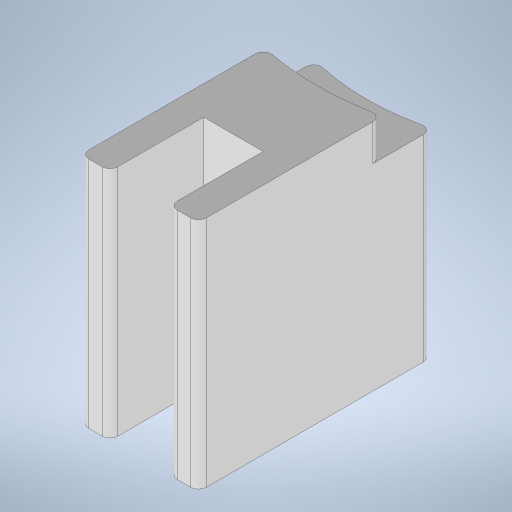
# Autodesk Inventor part: zigu2
Saved by Autodesk Inventor 2024.3 (Build 283343010, 343A)
## iProperties
Created: 2025-10-17
Part Number: zigu2
Material: 一般
Document SubType Name: Modeling
Designer: tanoue_kota
Density: 1 g/cm^3
Appearance: 既定
Author: tanoue_kota
Autodesk Inventor part; units mm, degrees
ref_plane "YZ Plane" through (0, 0, 0) normal (1, 0, 0) x (0, 1, 0)
ref_plane "XZ Plane" through (0, 0, 0) normal (0, 1, 0) x (-1, 0, 0)
ref_plane "XY Plane" through (0, 0, 0) normal (0, 0, 1) x (1, 0, 0)
sketch "スケッチ2" plane through (0, 0, 0) normal (0, 1, 0) x (-1, 0, 0)
  circle A0 centre (0, 0) radius 86.2565
  circle A1 centre (0, 0) radius 70
  circle A2 centre (0, 0) radius 57.5
  line L0 (0, 0) -> (0, 86.2565)
  line L1 (-14.9, 55.5359) -> (-14.9, 84.9598)
  line L2 (14.9, 55.5359) -> (14.9, 84.9598)
  line L3 (14.9, 84.9598) -> (-14.9, 84.9598)
  line L4 (-14.9, 84.9598) -> (-14.9, 115)
  line L5 (-14.9, 115) -> (14.9, 115)
  line L6 (14.9, 115) -> (14.9, 84.9598)
  line L7 (0, 115) -> (7.525, 115)
  line L8 (7.525, 115) -> (7.525, 91.2565)
  line L9 (7.525, 91.2565) -> (0, 91.2565)
  line L10 (0, 91.2565) -> (0, 115)
  line L11 (-7.525, 115) -> (-7.525, 91.2565)
  line L12 (-7.525, 91.2565) -> (0, 91.2565)
  dimension "d8" = 115
  dimension "d6" = 172.513
  dimension "d7" = 140
  dimension "d9" = 14.9
  dimension "d11" = 7.525
  dimension "d12" = 5
  dimension "d13" = 115
  constraints: 26 end point, 5 parallel, 4 coincident, 4 symmetric about line, 2 centre point, 2 horizontal, 2 perpendicular, 2 point on circle, 1 midpoint, 1 point on line, 1 vertical, 3 other
  measures "d6" diameter of A0
  measures "d7" diameter of A1
  measures "d9" distance between parallel lines of L0 L1
  measures "d11" distance of L8.end L9.end
  measures "d12" distance from line of point (0, 86.257) L9
  measures "d13" distance from line of point (0, 0) L5
extrude "押し出し2" add sketch "スケッチ2" along normal blind 59.1 contours L3 L0 A0 | L2 A1 L0 L3 | A0 L4 L5 L11 L12 L9 L8 L6 | L3 L0 A1 L1 | A0 L0 L3 | L2 A2 L0 A1 | A1 L0 A2 L1
sketch "スケッチ3" plane through (0, 59.1, 0) normal (0, 1, 0) x (1, 0, 0)
  circle A0 centre (0, 0) radius 70
  arc A1 (-14.9, -55.5359) -> (14.9, -55.5359) centre (0, 0) ccw projected
  circle A2 centre (0, 0) radius 57.5
  line L0 (-14.9, -55.5359) -> (-14.9, -68.3958)
  line L1 (14.9, -55.5359) -> (14.9, -68.3958)
  dimension "d16" = 140
  constraints: 4 end point, 2 coincident, 2 point on circle, 1 centre point, 1 parallel, 1 vertical, 3 other
  measures "d16" diameter of A0
extrude "押し出し3" cut sketch "スケッチ3" against normal blind 9.2 contours L0 A1 L1 A0
fillet "フィレット1" radius 2 8 edges at (-7.525, 29.55, 115) (7.525, 29.55, 115) (14.9, 29.55, 115) (-14.9, 29.55, 115) (14.9, 54.5, 68.3958) (-14.9, 54.5, 68.3958) (14.9, 24.95, 55.5359) (-14.9, 24.95, 55.5359)
